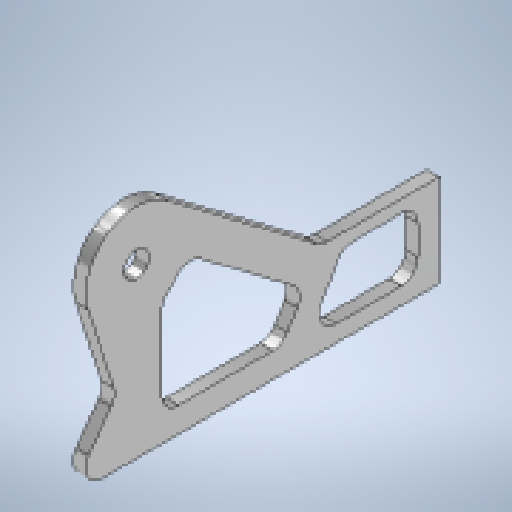
# Autodesk Inventor part: Upright
Saved by Autodesk Inventor 2023.4 (Build 274418000, 418)
## iProperties
Created: 2023-11-13
Part Number: Upright
Material: Aluminum 6061
Document SubType Name: Modeling
Designer: Nathan Cai
Density: 2.7 g/cm^3
Appearance: Aluminum - Flat
Mass: 57.2001 g
Surface Area: 121.868 cm^2
Volume: 21.1852 cm^3
Author: Nathan Cai
Autodesk Inventor part; units mm, degrees
ref_plane "YZ Plane" through (0, 0, 0) normal (1, 0, 0) x (0, 1, 0)
ref_plane "XZ Plane" through (0, 0, 0) normal (0, 1, 0) x (-1, 0, 0)
ref_plane "XY Plane" through (0, 0, 0) normal (0, 0, 1) x (1, 0, 0)
sketch "Sketch1" plane through (0, 0, 0) normal (1, 0, 0) x (0, 1, 0)
  circle A0 centre (0, 0) radius 4.7625
  line L0 (0, 0) -> (-63.5, 0) construction
  circle A1 centre (0, 0) radius 19.05
  line L1 (-5.715, 18.1725) -> (-63.5, 0)
  line L2 (-63.5, 0) -> (-63.5, -114.3)
  circle A2 centre (0, 0) radius 76.2 construction
  line L3 (-63.5, -114.3) -> (-28.575, -114.3)
  line L4 (-28.575, -114.3) -> (-28.575, -69.85)
  line L5 (-28.575, -69.85) -> (-63.5, -49.686)
  line L6 (-28.575, -69.85) -> (15.24, -11.43)
  line L7 (-39.6531, -63.4541) -> (-5.6963, -18.1784)
  line L8 (-53.975, -9.525) -> (-53.975, -55.1853)
  line L9 (-33.3375, -78.0989) -> (-63.5, -60.6846)
  line L10 (-33.3375, -78.0989) -> (-33.3375, -106.3625)
  line L11 (-33.3375, -106.3625) -> (-57.15, -106.3625)
  line L12 (-57.15, -106.3625) -> (-57.15, -64.3507)
  line L13 (-53.975, -9.525) -> (-52.0847, -9.525)
  line L14 (-52.0847, -9.525) -> (-16.4978, -9.525)
  line L15 (-63.5, 0) -> (-28.575, 0)
  line L16 (-28.575, 0) -> (-28.575, 25.4) construction
  line L17 (-28.575, 25.4) -> (-63.5, 25.4) construction
  line L18 (-63.5, 25.4) -> (-63.5, 0)
  line L19 (-28.575, 0) -> (-63.5, 25.4)
  point P0 (-39.1181, 7.6677)
  dimension "d0" = 9.525
  dimension "d1" = 63.5
  dimension "d2" = 38.1
  dimension "d3" = 114.3
  dimension "d4" = 152.4
  dimension "d5" = 34.925
  dimension "d6" = 44.45
  dimension "d7" = 60
  dimension "d9" = 12.7
  dimension "d10" = 9.525
  dimension "d11" = 9.525
  dimension "d12" = 7.9375
  dimension "d13" = 6.35
  dimension "d14" = 4.7625
  dimension "d17" = 9.525
  dimension "d19" = 34.925
  dimension "d20" = 25.4
  constraints: 40 end point, 6 parallel, 6 point on line, 4 point on circle, 3 centre point, 3 coincident, 3 horizontal, 3 perpendicular, 2 tangent, 1 vertical
  measures "d0" diameter of A0
  measures "d1" distance of L0.start L0.end
  measures "d2" diameter of A1
  measures "d3" distance of L0.end L2.end
  measures "d4" diameter of A2
  measures "d5" distance of L2.end L3.end
  measures "d6" distance of L3.end L4.end
  measures "d7" angle of L2 L5
  measures "d9" distance between parallel lines of L6 L7
  measures "d10" distance between parallel lines of L2 L8
  measures "d11" distance between parallel lines of L5 L9
  measures "d12" distance between parallel lines of L3 L11
  measures "d13" distance between parallel lines of L2 L12
  measures "d14" distance between parallel lines of L4 L10
  measures "d17" distance from line of L0 L8.start
  measures "d19" distance of L17.end L16.end
  measures "d20" distance of L16.end L15.end
extrude "Extrusion1" add sketch "Sketch1" along normal blind 4.7625 contours A1 | A1 L14 L13 L8 L5 L2 L15 L19 L1 | L6 L5 L7 A1 | L19 L15 L1 | L1 L18 L19 | L4 L3 L2 L5
fillet "Fillet1" radius 6.35 10 edges at (2.3813, -5.6963, -18.1784) (2.3813, -16.4978, -9.525) (2.3813, -39.6531, -63.4541) (2.3813, -53.975, -9.525) (2.3813, -53.975, -55.1853) (2.3813, -57.15, -64.3507) (2.3813, -33.3375, -78.0989) (2.3813, -33.3375, -106.3625) (2.3813, -57.15, -106.3625) (2.3813, -28.575, -69.85)
fillet "Fillet2" radius 6.35 2 edges at (2.3813, -63.5, 25.4) (2.3813, -39.1181, 7.6677)
sketch "Sketch2" plane through (4.7625, 0, 0) normal (1, 0, 0) x (0, 0, -1)
  circle A0 centre (0, 0) radius 4.7625 projected
  circle A1 centre (0, 0) radius 11.1125
  dimension "d24" = 22.225
  constraints: 1 centre point, 1 coincident
  measures "d24" diameter of A1
equation "\"d9\" = d8"
equation "\"d8\" = 12.7"
body "Solid1"
